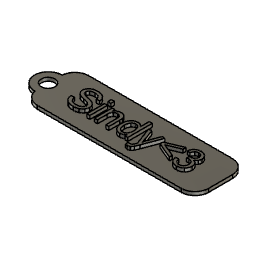
Sindy Name Tag (Autodesk Fusion 360 design; units mm, degrees)
Autodesk Fusion 360 part; units mm, degrees
note: some values were not read from the file. Set by a fixed rule: which sketch regions a step uses.
sketch "Sketch1" plane through (0, 0, 0) normal (0, 0, 1) x (1, 0, 0)
  line L0 (4, 15) -> (46, 15)
  line L1 (50, 11) -> (50, 4)
  line L2 (46, 0) -> (4, 0)
  line L3 (0, 4) -> (0, 11)
  arc A0 (4, 15) -> (0, 11) centre (4, 11) ccw
  arc A1 (50, 11) -> (46, 15) centre (46, 11) ccw
  arc A2 (46, 0) -> (50, 4) centre (46, 4) ccw
  arc A3 (0, 4) -> (4, 0) centre (4, 4) ccw
  circle A4 centre (-0.1026, 7.2545) radius 2
  circle A5 centre (-0.0572, 7.2463) radius 4
  dimension "d1" = 4
  dimension "d2" = 4
  dimension "d3" = 8
  constraint horizontal L0
  constraint vertical L1
  constraint horizontal L2
  constraint vertical L3
  constraint tangent L0 A0
  constraint tangent L3 A0
  constraint tangent L0 A1
  constraint tangent L1 A1
  constraint equal A0 A1
  constraint tangent L1 A2
  constraint tangent L2 A2
  constraint equal A0 A2
  constraint tangent L2 A3
  constraint tangent L3 A3
  constraint equal A0 A3
  measures "d1" radius of A0
  measures "d2" diameter of A4
  measures "d3" diameter of A5
extrude "Extrude1" add sketch "Sketch1" along normal blind 1 contours L0 L1 L2 A0 A1 A2 A3 A5 | L3 A0 A3 A4 A5 | L3 A0 A3 A4 A5
sketch "Sketch2" plane through (0, 0, 1) normal (0, 0, 1) x (-1, 0, 0)
  circle A0 centre (0.1026, -7.2545) radius 2
  arc A1 (-50, -11) -> (-46, -15) centre (-46, -11) ccw
  line L0 (-46, -15) -> (-4, -15)
  arc A2 (-4, -15) -> (-0.0076, -11.2458) centre (-4, -11) ccw
  arc A3 (-0.0076, -11.2458) -> (-0.0713, -3.2483) centre (0.0572, -7.2463) ccw
  arc A4 (-0.0713, -3.2483) -> (-4, 0) centre (-4, -4) ccw
  line L1 (-4, 0) -> (-46, 0)
  arc A5 (-46, 0) -> (-50, -4) centre (-46, -4) ccw
  line L2 (-50, -4) -> (-50, -11)
  line L3 (-7.4765, -1.9632) -> (-42.9892, -1.9632) construction
  line L4 (-42.9892, -1.9632) -> (-42.9892, -11.9632) construction
  line L5 (-42.9892, -11.9632) -> (-7.4765, -11.9632) construction
  line L6 (-7.4765, -11.9632) -> (-7.4765, -1.9632) construction
  text T0 "Sindy<3" font "Arial" height 10 align ink ink in box 0 x 0 at (-7.4865, -1.9832) x (-1, 0) y (0, -1) spacing 1 height is em
  constraint perpendicular L3 L4
  constraint parallel L3 L5
  constraint parallel L4 L6
extrude "Extrude2" add sketch "Sketch2" along normal blind 1 text T0
